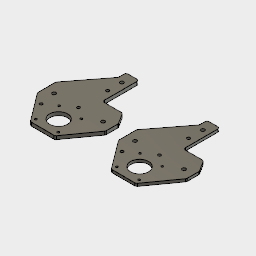
X_Motor_Bracket_v2 (Autodesk Fusion 360 design; units mm, degrees)
Autodesk Fusion 360 part; units mm, degrees
sketch "Sketch1" plane through (0, 0, 0) normal (0, 1, 0) x (1, 0, 0)
  line L0 (-42.1826, -28.8614) -> (-13.0043, -67.7642)
  line L1 (53.0032, -27.598) -> (24.1261, -67.7738)
  line L2 (53.1034, -7.7852) -> (44.1969, 6.3117)
  line L3 (-42.2998, -0.9941) -> (-4.6185, 48.1926)
  line L4 (-4, 50.0171) -> (-4, 57)
  circle A0 centre (5, -45.5) radius 12.8153
  circle A1 centre (5, -17) radius 2
  circle A2 centre (4.9576, 24.5785) radius 2.1213
  circle A3 centre (5, 45) radius 2.5
  circle A4 centre (40, -17) radius 2.5
  circle A5 centre (-30, -17) radius 2.5
  circle A6 centre (-11.0748, -28.8383) radius 1.5
  circle A7 centre (21, -29) radius 1.5
  circle A8 centre (-11, -62) radius 1.5
  circle A9 centre (21.0748, -62.1617) radius 1.5
  circle A10 centre (-26.2214, -39.364) radius 2
  line L5 (-10.6098, -68.9642) -> (21.6846, -69.0228)
  line L6 (53.5672, -25.8471) -> (53.5672, -9.3876)
  line L7 (41.6607, 7.7093) -> (17.4638, 7.7093)
  line L8 (-42.9182, -2.8353) -> (-42.7826, -27.0781)
  line L9 (-1, 60) -> (11.4638, 60)
  line L10 (14.4638, 57) -> (14.4638, 10.7093)
  arc A11 (14.4638, 57) -> (11.4638, 60) centre (11.4638, 57) ccw
  arc A12 (-1, 60) -> (-4, 57) centre (-1, 57) ccw
  arc A13 (-4.6185, 48.1926) -> (-4, 50.0171) centre (-7, 50.0171) ccw
  arc A14 (-42.2998, -0.9941) -> (-42.9182, -2.8353) centre (-39.9183, -2.8185) ccw
  arc A15 (-42.7826, -27.0781) -> (-42.1826, -28.8614) centre (-39.7827, -27.0614) ccw
  arc A16 (-13.0043, -67.7642) -> (-10.6098, -68.9642) centre (-10.6044, -65.9642) ccw
  arc A17 (21.6846, -69.0228) -> (24.1261, -67.7738) centre (21.6901, -66.0228) ccw
  arc A18 (53.0032, -27.598) -> (53.5672, -25.8471) centre (50.5672, -25.8471) ccw
  arc A19 (53.5672, -9.3876) -> (53.1034, -7.7852) centre (50.5672, -9.3876) ccw
  arc A20 (44.1969, 6.3117) -> (41.6607, 7.7093) centre (41.6607, 4.7093) ccw
  arc A21 (14.4638, 10.7093) -> (17.4638, 7.7093) centre (17.4638, 10.7093) ccw
  dimension "d1" = 4
  dimension "d2" = 5
  dimension "d3" = 5
  dimension "d4" = 5
  dimension "d5" = 3
  dimension "d6" = 3
  dimension "d7" = 3
  dimension "d8" = 3
  dimension "d9" = 4
  dimension "d13" = 3
  measures "d1" diameter of A1
  measures "d2" diameter of A4
  measures "d3" diameter of A3
  measures "d4" diameter of A5
  measures "d5" diameter of A6
  measures "d6" diameter of A7
  measures "d7" diameter of A8
  measures "d8" diameter of A9
  measures "d9" diameter of A10
  measures "d13" radius of A11
extrude "Extrude2" add sketch "Sketch1" along normal blind 5 makes body 1
copy_body "CopyPasteBodies1" bodies 1 makes body 2
move_body "Move1" bodies 2 to x (1, 0, 0) y (0, 1, 0) z (0, 0, 1) at (110, 0, 0)
move_face "OffsetFaces1" offset -1 1 faces at (102.9763, 5, 2.5254) on bodies 2
scale "Scale1" factor 0.95 about (113, 4, 17) bodies 2
scale "Scale2" factor 0.95 about (3, 5, 17) bodies 1
named bodies: "5mm", "4mm"
